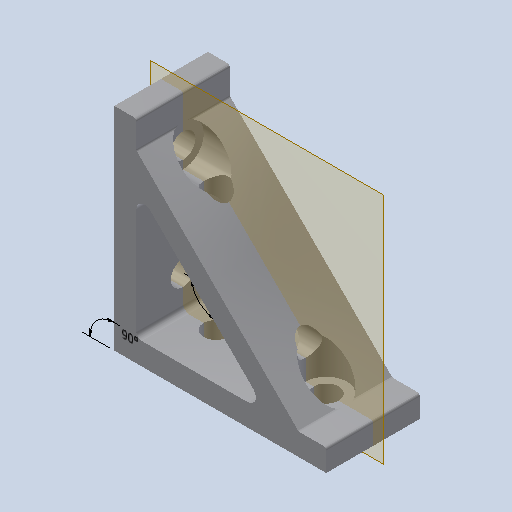
# Autodesk Inventor part: 20-102
Saved by Autodesk Inventor 2022 (Build 260153000, 153)
## iProperties
Created: 2004-11-12
Part Number: 20-102
Material: Alluminio - 6061
Document SubType Name: Modeling
Designer: Chapin
Manufacturer: Standard
Standards Organization: Custom
Mass: 149.365 g
Surface Area: 189.415 cm^2
Volume: 55.3203 cm^3
Density: 2.7 g/cm^3
Appearance: Alluminio - Piatto
LastFilename: Not Set
Title: GUSSET PROFILE 80
Author: Chapin
Autodesk Inventor part; units mm, degrees
ref_plane "YZ Plane" through (0, 0, 0) normal (1, 0, 0) x (0, 1, 0)
sketch "Sketch1" plane through (0, 0, 0) normal (0, 0, 1) x (1, 0, 0)
  line L0 (-38.481, 38.481) -> (38.481, 38.481)
  line L1 (38.481, 38.481) -> (38.481, -38.481)
  line L2 (38.481, -38.481) -> (-38.481, -38.481)
  line L3 (-38.481, -38.481) -> (-38.481, 38.481)
  point P0 (0, 0)
  dimension "d0" = 76.962
  dimension "d1" = 76.962
  dimension "d2" = 38.481
  dimension "d3" = 38.481
  constraints: 8 end point, 2 parallel, 1 horizontal, 1 perpendicular
  measures "d0" distance of L0.start L0.end
  measures "d1" distance of L2.end L0.start
  measures "d2" distance from line of point (0, 0) L3
  measures "d3" distance from line of point (0, 0) L0
extrude "Extrusion1" add sketch "Sketch1" against normal blind 34
sketch "Sketch2" plane through (0, 0, 0) normal (0, 0, 1) x (1, 0, 0)
  line L0 (-38.481, 38.481) -> (38.481, 38.481) projected
  line L1 (-38.481, -38.481) -> (-38.481, 38.481) projected
  line L2 (38.481, -38.481) -> (-38.481, -38.481) projected
  line L3 (38.481, 38.481) -> (38.481, -38.481) projected
  line L4 (-30.481, 38.481) -> (-30.481, 28.481)
  line L5 (-30.481, 28.481) -> (28.481, -30.481)
  line L6 (28.481, -30.481) -> (38.481, -30.481)
  line L7 (-30.481, 17.1673) -> (-30.481, -30.481)
  line L8 (-30.481, -30.481) -> (17.1673, -30.481)
  line L9 (17.1673, -30.481) -> (-30.481, 17.1673)
  dimension "d6" = 8
  dimension "d7" = 8
  dimension "d8" = 10
  dimension "d10" = 135
  dimension "d11" = 8
  constraints: 12 end point, 2 collinear, 2 parallel, 2 perpendicular, 2 point on line, 1 horizontal
  measures "d6" distance between parallel lines of L1 L4
  measures "d7" distance between parallel lines of L2 L6
  measures "d8" distance of L4.start L4.end
  measures "d10" angle of L5 L4
  measures "d11" distance between parallel lines of L5 L9
extrude "Extrusion2" cut sketch "Sketch2" against normal through all contours L0 L3 L6 L5 L4 | L9 L8 L7
fillet "Fillet1" radius 2 1 edges at (-30.481, -30.481, -17)
fillet "Fillet1" radius 1 4 edges at (-30.481, 38.481, -17) (-30.481, 28.481, -17) (28.481, -30.481, -17) (38.481, -30.481, -17)
fillet "Fillet1" radius 3 2 edges at (-30.481, 17.1673, -17) (17.1673, -30.481, -17)
sketch "Sketch3" plane through (-38.481, -38.481, 0) normal (-1, 0, 0) x (0, 0, 1)
  line L0 (0, 0) -> (-34, 0) projected
  line L1 (0, 0) -> (0, 76.962) projected
  point P0 (-17, 60)
  point P1 (-17, 20)
  dimension "d17" = 17
  dimension "d18" = 20
  dimension "d19" = 40
  constraints: 1 vertical alignment
  measures "d17" distance from line of L1 point (-17, 60)
  measures "d18" distance from line of L0 point (-17, 20)
  measures "d19" distance of point (-17, 60) point (-17, 20)
hole "Hole1" at (-38.481, 21.519, -17) at (-38.481, -18.481, -17) direction (1, 0, 0) diameter 9 end through all
sketch "Sketch4" plane through (-38.481, -38.481, 0) normal (0, -1, 0) x (1, 0, 0)
  line L0 (0, -34) -> (76.962, -34) projected
  line L1 (0, 0) -> (0, -34) projected
  point P0 (20, -17)
  point P1 (60, -17)
  dimension "d27" = 17
  dimension "d28" = 20
  dimension "d29" = 40
  constraints: 1 horizontal alignment
  measures "d27" distance from line of L0 point (20, -17)
  measures "d28" distance from line of L1 point (20, -17)
  measures "d29" distance of point (60, -17) point (20, -17)
hole "Hole2" at (-18.481, -38.481, -17) at (21.519, -38.481, -17) direction (0, 1, 0) diameter 9 end through all
ref_plane "Work Plane1" through (-30.481, -38.481, 0) normal (-1, 0, 0) x (0, 0, 1)
ref_plane "Work Plane2" through (-38.481, -30.481, 0) normal (0, -1, 0) x (1, 0, 0)
sketch "Sketch5" plane through (-30.481, -38.481, 0) normal (-1, 0, 0) x (0, 0, 1)
  arc A0 (-13.2711, 57.481) -> (-20.7289, 57.481) centre (-17, 60) ccw projected
  circle A1 centre (-17, 60) radius 4.5 projected
  circle A2 centre (-17, 60) radius 7.5
  dimension "d39" = 15
  constraints: 1 centre point, 1 coincident, 1 horizontal alignment
  measures "d39" diameter of A2
extrude "Extrusion3" cut sketch "Sketch5" against normal through all
sketch "Sketch6" plane through (-38.481, -30.481, 0) normal (0, -1, 0) x (1, 0, 0)
  arc A0 (57.481, -20.7289) -> (57.481, -13.2711) centre (60, -17) ccw projected
  circle A1 centre (60, -17) radius 4.5 projected
  circle A2 centre (60, -17) radius 7.5
  dimension "d42" = 15
  constraints: 1 centre point, 1 coincident, 1 vertical alignment
  measures "d42" diameter of A2
extrude "Extrusion4" cut sketch "Sketch6" against normal through all
ref_plane "OffsetPlane" through (0, 0, -17) normal (0, 0, 1) x (1, 0, 0)
equation "\"d2\" = 0.5 * d0"
equation "\"d3\" = 0.5 * d1"
